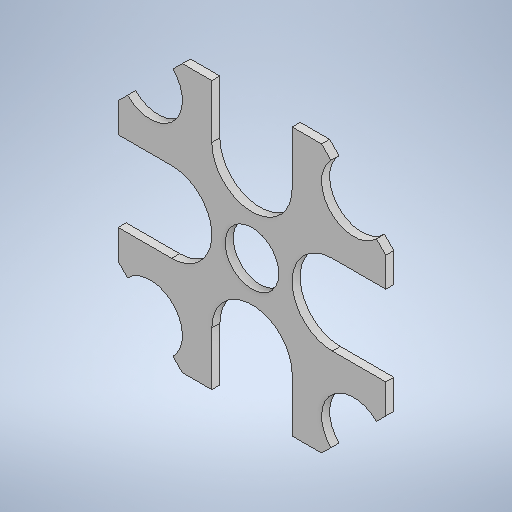
# Autodesk Inventor part: Desafio 1 - MASA - Inventor
Saved by Autodesk Inventor 2025.1 (Build 291241000, 241)
## iProperties
Created: 2025-05-16
Part Number: Desafio 1 - MASA - Inventor
Material: Generic
Document SubType Name: Modeling
Designer: Aluno
Density: 1 g/cm^3
Appearance: Default
Author: Aluno
Autodesk Inventor part; units mm, degrees
ref_plane "YZ Plane" through (0, 0, 0) normal (1, 0, 0) x (0, 1, 0)
ref_plane "XZ Plane" through (0, 0, 0) normal (0, 1, 0) x (-1, 0, 0)
ref_plane "XY Plane" through (0, 0, 0) normal (0, 0, 1) x (1, 0, 0)
sketch "Sketch1" plane through (0, 0, 0) normal (0, 0, 1) x (1, 0, 0)
  circle A0 centre (0, 0) radius 10
  arc A1 (-30, -15) -> (-30, 15) centre (-30, 0) ccw
  arc A2 (30, 15) -> (30, -15) centre (30, 0) ccw
  arc A3 (-15, 30) -> (15, 30) centre (0, 30) ccw
  arc A4 (15, -30) -> (-15, -30) centre (0, -30) ccw
  line L0 (-30, 15) -> (-50, 15)
  line L1 (-30, -15) -> (-50, -15)
  line L2 (-15, -30) -> (-15, -50)
  line L3 (15, -30) -> (15, -50)
  line L4 (30, 15) -> (50, 15)
  line L5 (30, -15) -> (50, -15)
  line L6 (-15, 30) -> (-15, 50)
  line L7 (15, 30) -> (15, 50)
  line L8 (-50, -26) -> (-50, -15)
  line L9 (-50, 15) -> (-50, 26)
  line L10 (50, 26) -> (50, 15)
  line L11 (-26, 50) -> (-15, 50)
  arc A5 (-46.4853, 29.5147) -> (-29.5147, 46.4853) centre (-38, 38) ccw
  arc A6 (29.5147, 46.4853) -> (46.4853, 29.5147) centre (38, 38) ccw
  arc A7 (-29.5147, -46.4853) -> (-46.4853, -29.5147) centre (-38, -38) ccw
  arc A8 (46.4853, -29.5147) -> (29.5147, -46.4853) centre (38, -38) ccw
  line L12 (-29.5147, 46.4853) -> (-26, 50)
  line L13 (-46.4853, 29.5147) -> (-50, 26)
  line L14 (46.4853, 29.5147) -> (50, 26)
  line L15 (26, 50) -> (29.5147, 46.4853)
  line L16 (-29.5147, -46.4853) -> (-26, -50)
  line L17 (-50, -26) -> (-46.4853, -29.5147)
  line L18 (46.4853, -29.5147) -> (50, -26)
  line L19 (29.5147, -46.4853) -> (26, -50)
  line L20 (15, 50) -> (26, 50)
  line L21 (26, -50) -> (15, -50)
  line L22 (50, -15) -> (50, -26)
  line L23 (-15, -50) -> (-26, -50)
  dimension "d1" = 20
  dimension "d2" = 30
  dimension "d4" = 30
  dimension "d5" = 30
  dimension "d6" = 30
  dimension "d7" = 24
  dimension "d8" = 24
  dimension "d9" = 24
  dimension "d10" = 24
  dimension "d11" = 20
  dimension "d12" = 20
  dimension "d13" = 20
  constraints: 48 end point, 16 point on circle, 12 point on line, 10 perpendicular, 9 centre point, 9 coincident, 4 tangent, 3 equal length
  measures "d1" diameter of A0
  measures "d2" diameter of A1
  measures "d4" diameter of A2
  measures "d5" diameter of A3
  measures "d6" diameter of A4
  measures "d7" diameter of A5
  measures "d8" diameter of A6
  measures "d9" diameter of A7
  measures "d10" diameter of A8
  measures "d11" vertical distance of point (0, 30) L7.end
  measures "d12" horizontal distance of L0.end point (-30, 0)
  measures "d13" vertical distance of L2.end point (0, -30)
extrude "Extrusion1" add sketch "Sketch1" along normal blind 3
body "Solid1"
